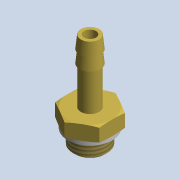
# Autodesk Inventor part: 15631 N-1/4-P-6-MS
Saved by Autodesk Inventor 2021 (Build 250183000, 183)
## iProperties
Part Number: 15631 N-1/4-P-6-MS
Material: Genérico
Catalog Web Link: www.cadenas.de
Description: N-..-P-..-MS-barbed hose fitting
Vendor: FESTO
Document SubType Name: Modeling
Designer: partserver
Manufacturer: FESTO
Mass: 2.88949 g
Surface Area: 21.7368 cm^2
Volume: 2.88949 cm^3
Density: 1 g/cm^3
Appearance: PSOLRGB-229-204-89
Category: PARTsolutions
Company: FESTO
PSOL_IDENT_0: {$CADENAS_DATA\23d-libs\festo\parts\n\n\n_p_ms.prj},182 {VTYP=3D},{NB=15631 N-1/4-P-6-MS},{LINA=1563
PSOL_IDENT_1: 1 N-1/4-P-6-MS},{NN=N-..-P-..-MS},{DATE=27.04.2020 09:06:56},{GEOMDATE=04.09.2015 09:36:03},{VERSION=
PSOL_IDENT_2: },{LINEID=20},{WBVAR=},{WBNUMERIC=}  {NB=15631 N-1/4-P-6-MS},{LINA=15631 N-1/4-P-6-MS},{KT=DUMMY},{T
PSOL_IDENT_3: NR=15631},{TYP=N-1/4-P-6-MS},{L=37.100},{L1=7.000},{L2=24.100},{B=6.000},{D1=G1/4},{D1NDM=13.157},{D
PSOL_IDENT_4: 1KDM=11.445},{D2=7.000},{NW=4.500},{SW=17.000}
NB: 15631 N-1/4-P-6-MS
NN: N-..-P-..-MS
NT: barbed hose fitting
NBSYN: $TNR. $TYP.
LINA: 15631 N-1/4-P-6-MS
CATALOG: Festo
TNR: 15631
TYP: N-1/4-P-6-MS
L: 37.1
L1: 7
L2: 24.1
B: 6
D1: G1/4
D2: 7
NW: 4.5
SW: 17
SUPPLIER: FESTO
ARTICLENO: 15631 N-1/4-P-6-MS
BOMINFO: 15631 N-1/4-P-6-MS
CREATOR: CADENAS GmbH
Title: 15631 N-1/4-P-6-MS
Author: Cadenas PARTsolutions
Comments: barbed hose fitting
Autodesk Inventor part; units mm, degrees
sketch "Skizze_1" plane through (0, 0, 0) normal (1, 0, 0) x (0, 1, 0)
  line L0 (0, -37.1) -> (0, 0)
  line L1 (0, 0) -> (5.7225, 0)
  line L2 (5.7225, 0) -> (6.5785, -0.856)
  line L3 (6.5785, -0.856) -> (6.5785, -6)
  line L4 (6.5785, -6) -> (8.5, -6)
  line L5 (8.5, -6) -> (8.5, -7.4)
  line L6 (8.5, -7.4) -> (10.2, -7.8555)
  line L7 (10.2, -7.8555) -> (10.2, -12.5445)
  line L8 (10.2, -12.5445) -> (8.5, -13)
  line L9 (8.5, -13) -> (3.5, -13)
  line L10 (3.5, -13) -> (3.5, -27.46)
  line L11 (3.5, -27.46) -> (4, -27.46)
  line L12 (4, -27.46) -> (3.5, -32.28)
  line L13 (3.5, -32.28) -> (4, -32.28)
  line L14 (4, -32.28) -> (3.5, -37.1)
  line L15 (3.5, -37.1) -> (0, -37.1)
  line L16 (0, -37.1) -> (0, 0)
  constraints: 34 end point
revolve "Revolution1" add sketch "Skizze_1" angle 360 about axis through (0, 0, -37.1) along (0, 0, -1)
thread "Thread1" size "G13.157x1.337" designation "G 1/4" class "A" standard "ISO Pipe Threads" length 4.394
sketch "Sketch2" plane through (0, 0, 0) normal (0, 0, 1) x (1, 0, 0)
  point P0 (0, 0)
hole "Hole1" at (0, 0, 0) direction (0, 0, -1) diameter 4.5 depth 37.1 countersink diameter 6.8094 countersink angle 60
sketch "Skizze_3" plane through (0, 0, 0) normal (0, 0, 1) x (1, 0, 0)
  line L0 (-17, -17) -> (17, -17)
  line L1 (17, -17) -> (17, 17)
  line L2 (17, 17) -> (-17, 17)
  line L3 (-17, 17) -> (-17, -17)
  line L4 (-8.5, -4.9075) -> (0, -9.815)
  line L5 (0, -9.815) -> (8.5, -4.9075)
  line L6 (8.5, -4.9075) -> (8.5, 4.9075)
  line L7 (8.5, 4.9075) -> (0, 9.815)
  line L8 (0, 9.815) -> (-8.5, 4.9075)
  line L9 (-8.5, 4.9075) -> (-8.5, -4.9075)
  constraints: 20 end point
extrude "Extrusion1" cut sketch "Skizze_3" against normal blind 13
ref_plane "ANBAU_STD_XY" through (0, 0, -6) normal (0, 0, -1) x (1, 0, 0)
ref_plane "ANBAU_STD_YZ" through (0, 0, -6) normal (1, 0, 0) x (0, -1, 0)
ref_plane "ANBAU_STD_ZX" through (0, 0, -6) normal (0, -1, 0) x (0, 0, -1)
body "Solid1"
